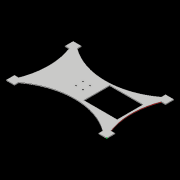
# Autodesk Inventor part: TopV3
Saved by Autodesk Inventor 2019 (Build 230136000, 136)
## iProperties
Created: 2021-09-17
Part Number: TopV3
Material: Generic
Document SubType Name: Modeling
Designer: timmy
Density: 1 g/cm^3
Appearance: Default
Author: timmy
Autodesk Inventor part; units mm, degrees
ref_plane "YZ Plane" through (0, 0, 0) normal (1, 0, 0) x (0, 1, 0)
ref_plane "XZ Plane" through (0, 0, 0) normal (0, 1, 0) x (-1, 0, 0)
ref_plane "XY Plane" through (0, 0, 0) normal (0, 0, 1) x (1, 0, 0)
sketch "Sketch1" plane through (0, 0, 0) normal (0, 1, 0) x (-1, 0, 0)
  line L0 (0, 0) -> (914.4, 0)
  line L1 (914.4, 0) -> (914.4, -609.6)
  line L2 (914.4, -609.6) -> (0, -609.6)
  line L3 (0, -609.6) -> (0, 0)
  line L4 (0, -609.6) -> (76.2, -609.6)
  line L5 (76.2, -609.6) -> (76.2, -533.4)
  line L6 (76.2, -533.4) -> (0, -533.4)
  line L7 (0, -533.4) -> (0, -609.6)
  line L8 (0, 0) -> (76.2, 0)
  line L9 (76.2, 0) -> (76.2, -76.2)
  line L10 (76.2, -76.2) -> (0, -76.2)
  line L11 (0, -76.2) -> (0, 0)
  line L12 (914.4, -609.6) -> (838.2, -609.6)
  line L13 (838.2, -609.6) -> (838.2, -533.4)
  line L14 (838.2, -533.4) -> (914.4, -533.4)
  line L15 (914.4, -533.4) -> (914.4, -609.6)
  line L16 (914.4, 0) -> (838.2, 0)
  line L17 (838.2, 0) -> (838.2, -76.2)
  line L18 (838.2, -76.2) -> (914.4, -76.2)
  line L19 (914.4, -76.2) -> (914.4, 0)
  arc A0 (838.2, -571.5) -> (76.2, -571.5) centre (457.2, -1079.5) ccw
  arc A1 (76.2, -38.1) -> (838.2, -38.1) centre (457.2, 469.9) ccw
  arc A2 (876.3, -76.2) -> (876.3, -533.4) centre (1468.7247, -304.8) ccw
  arc A3 (38.1, -533.4) -> (38.1, -76.2) centre (-554.3247, -304.8) ccw
  dimension "d17" = 609.6
  dimension "d18" = 76.2
  dimension "d19" = 76.2
  dimension "d20" = 76.2
  dimension "d21" = 76.2
  dimension "d22" = 76.2
  dimension "d23" = 76.2
  dimension "d24" = 76.2
  dimension "d25" = 76.2
  dimension "d26" = 635
  dimension "d27" = 635
  dimension "d28" = 635
  dimension "d29" = 635
  constraints: 40 end point, 10 parallel, 8 midpoint, 8 point on circle, 5 horizontal, 5 perpendicular, 4 centre point
  measures "d17" distance of L0.end L1.end
  measures "d18" distance of L6.end L5.end
  measures "d19" distance of L5.end L4.end
  measures "d20" distance of L9.end L10.end
  measures "d21" distance of L8.end L9.end
  measures "d22" distance of L13.end L14.end
  measures "d23" distance of L12.end L13.end
  measures "d24" distance of L18.end L17.end
  measures "d25" distance of L17.end L16.end
  measures "d26" radius of A0
  measures "d27" radius of A1
  measures "d28" radius of A2
  measures "d29" radius of A3
extrude "Extrusion2" add sketch "Sketch1" along normal blind 6.35 contours L0 L9 L10 L3 | L0 L1 L18 L17 | A1 L17 L18 A2 L14 L13 A0 L5 L6 A3 L10 L9 | L6 L5 L2 L3 | L1 L2 L13 L14
sketch "Sketch2" plane through (0, 6.35, 0) normal (0, 1, 0) x (1, 0, 0)
  arc A0 (-76.2, 38.1) -> (-838.2, 38.1) centre (-457.2, -469.9) ccw projected
  arc A1 (-838.2, 571.5) -> (-76.2, 571.5) centre (-457.2, 1079.5) ccw projected
  line L0 (-457.2, 304.8) -> (-457.2, 241.3)
  line L1 (-457.2, 241.3) -> (-584.2, 241.3)
  line L2 (-584.2, 241.3) -> (-584.2, 368.3)
  line L3 (-584.2, 368.3) -> (-457.2, 368.3)
  line L4 (-457.2, 368.3) -> (-457.2, 241.3)
  line L5 (-584.2, 304.8) -> (-520.7, 368.3) construction
  line L6 (-520.7, 368.3) -> (-457.2, 304.8) construction
  line L7 (-552.45, 336.55) -> (-488.95, 336.55) construction
  line L8 (-584.2, 304.8) -> (-520.7, 241.3) construction
  line L9 (-457.2, 304.8) -> (-520.7, 241.3) construction
  line L10 (-552.45, 273.05) -> (-488.95, 273.05) construction
  circle A2 centre (-552.45, 273.05) radius 4.5 construction
  circle A3 centre (-488.95, 273.05) radius 4.5 construction
  circle A4 centre (-488.95, 336.55) radius 4.5 construction
  circle A5 centre (-552.45, 336.55) radius 4.5 construction
  point P0 (0, 0)
  dimension "d35" = 9
  dimension "d36" = 9
  dimension "d37" = 9
  dimension "d38" = 9
  constraints: 22 end point, 7 midpoint, 4 centre point, 4 coincident, 3 perpendicular, 2 parallel, 1 horizontal
  measures "d35" diameter of A2
  measures "d36" diameter of A3
  measures "d37" diameter of A4
  measures "d38" diameter of A5
hole "Hole1" at (-552.45, 6.35, -273.05) at (-552.45, 6.35, -336.55) at (-488.95, 6.35, -336.55) at (-488.95, 6.35, -273.05) direction (0, -1, 0) diameter 10.5918 end through all thread size "1/2-13 UNC" class "2B" standard "ANSI Unified Screw Threads"
sketch "Sketch3" plane through (0, 6.35, 0) normal (0, 1, 0) x (1, 0, 0)
  point P0 (0, 0)
sketch "Sketch4" plane through (0, 6.35, 0) normal (0, 1, 0) x (1, 0, 0)
  line L0 (-401.2293, 193.7971) -> (-99.5943, 193.7971)
  line L1 (-99.5943, 193.7971) -> (-99.5943, 428.1144)
  line L2 (-99.5943, 428.1144) -> (-401.2293, 428.1144)
  line L3 (-401.2293, 428.1144) -> (-401.2293, 193.7971)
  point P0 (0, 0)
  constraints: 8 end point, 2 parallel, 1 horizontal, 1 perpendicular
extrude "Extrusion3" cut sketch "Sketch4" against normal blind 6.35
body "Solid2"
